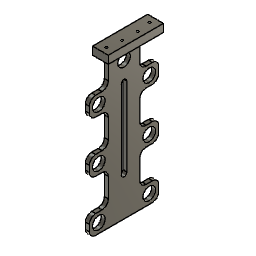
Riel Versión 3 v1 (Autodesk Fusion 360 design; units mm, degrees)
Autodesk Fusion 360 part; units mm, degrees
sketch "Boceto1" plane through (0, 0, 0) normal (0, 0, 1) x (1, 0, 0)
  line L0 (0, 0) -> (60, 0)
  line L1 (60, 0) -> (60, 40)
  line L2 (60, 40) -> (0, 40)
  line L3 (0, 40) -> (0, 0)
  line L4 (0, 0) -> (0, 10)
  line L5 (0, 40) -> (0, 30)
  line L6 (0, 30) -> (60, 30)
  line L7 (0, 10) -> (60, 10)
  line L8 (0, 30) -> (10, 30)
  line L9 (10, 40) -> (10, 0)
  line L10 (60, 40) -> (50, 40)
  line L11 (50, 40) -> (50, 0)
  circle A0 centre (5, 35) radius 2.5
  circle A1 centre (5, 5) radius 2.5
  circle A2 centre (55, 35) radius 2.5
  circle A3 centre (55, 5) radius 2.5
  line L12 (10, 10) -> (10, 9)
  line L13 (10, 9) -> (50, 9)
  line L14 (50, 30) -> (50, 31)
  line L15 (50, 31) -> (10, 31)
  line L16 (10, 0) -> (19, 0)
  line L17 (19, 9) -> (19, 0)
  line L18 (50, 0) -> (41, 0)
  line L19 (41, 0) -> (41, 9)
  line L20 (50, 31) -> (41, 31)
  line L21 (41, 31) -> (41, 40)
  line L22 (10, 31) -> (19, 31)
  line L23 (19, 31) -> (19, 40)
  line L24 (19, 9) -> (10, 0)
  line L25 (10, 9) -> (19, 0)
  circle A4 centre (14.5, 4.5) radius 2.5
  line L26 (19, 31) -> (10, 40)
  line L27 (50, 31) -> (41, 40)
  line L28 (50, 0) -> (41, 9)
  line L29 (50, 9) -> (41, 0)
  line L30 (50, 40) -> (41, 31)
  line L31 (19, 40) -> (10, 31)
  circle A5 centre (14.5, 35.5) radius 2.5
  circle A6 centre (45.5, 35.5) radius 2.5
  circle A7 centre (45.5, 4.5) radius 2.5
  line L32 (10, 9) -> (15, 9)
  line L33 (15, 9) -> (15, 31)
  line L34 (50, 9) -> (45, 9)
  line L35 (45, 9) -> (45, 31)
  dimension "d1" = 60
  dimension "d2" = 40
  dimension "d3" = 10
  dimension "d4" = 10
  dimension "d5" = 5
  dimension "d6" = 5
  dimension "d7" = 5
  dimension "d8" = 5
  dimension "d9" = 5
  dimension "d10" = 5
  dimension "d11" = 5
  dimension "d12" = 5
  constraint coincident L0.start L3.end
  constraint horizontal L0
  constraint perpendicular L0 L1
  constraint perpendicular L1 L2
  constraint perpendicular L0 L3
  constraint perpendicular L0 L4
  constraint perpendicular L2 L5
  constraint coincident L1 L6.end
  constraint perpendicular L1 L6
  constraint coincident L1 L7.end
  constraint perpendicular L1 L7
  constraint coincident L6 L8.end
  constraint coincident L2 L9.start
  constraint coincident L0 L9.end
  constraint perpendicular L0 L9
  constraint coincident L2 L10.end
  constraint perpendicular L7 L11
  constraint coincident L9 L12.start
  constraint coincident L7 L12.start
  constraint coincident L9 L12.end
  constraint coincident L11 L13.end
  constraint perpendicular L11 L13
  constraint coincident L11 L14.start
  constraint coincident L6 L14.start
  constraint coincident L11 L14.end
  constraint perpendicular L6 L14
  constraint coincident L9 L15.end
  constraint perpendicular L9 L15
  constraint coincident L0 L16.end
  constraint coincident L13 L17.start
  constraint perpendicular L16 L17
  constraint coincident L0 L18.end
  constraint perpendicular L11 L18
  constraint coincident L13 L19.end
  constraint perpendicular L13 L19
  constraint coincident L15 L20.end
  constraint coincident L2 L21.end
  constraint perpendicular L2 L21
  constraint coincident L15 L22.end
  constraint coincident L2 L23.end
  constraint perpendicular L2 L23
  constraint perpendicular L24 L25
  constraint midpoint L25 A4.centre
  constraint parallel L26 L27
  constraint parallel L27 L28
  constraint perpendicular L28 L29
  constraint midpoint L26 A5.centre
  constraint midpoint L30 A6.centre
  constraint midpoint L28 A7.centre
  constraint coincident L13 L32.end
  constraint perpendicular L9 L32
  constraint coincident L22 L33.end
  constraint coincident L13 L34.end
  constraint perpendicular L11 L34
  constraint coincident L20 L35.end
  measures "d1" distance of L0.start L0.end
  measures "d2" distance of L0.end L1.end
  measures "d3" distance of L0.start L4.end
  measures "d4" distance of L2.end L5.end
  measures "d5" diameter of A0
  measures "d6" diameter of A1
  measures "d7" diameter of A2
  measures "d8" diameter of A3
  measures "d9" diameter of A4
  measures "d10" diameter of A5
  measures "d11" diameter of A6
  measures "d12" diameter of A7
extrude "Extruir3" add sketch "Boceto1" along normal blind 20 contours L0 L3 L4 L7 L9 L12 | L0 L16 L24 L25 A4 | L9 L24 L25 A4 | L3 L6 L7 L8 L9 | L0 L13 L17 L19 | L17 L24 L25 A4 | L7 L9 L12 L13 L32 L33 | L13 L24 L25 A4 L32 | L2 L3 L5 L6 L8 L9 | L6 L7 L9 L33 | L0 L18 L28 L29 A7 | L19 L28 L29 A7 | L6 L9 L15 L22 L33 | L0 L1 L7 L11 | L11 L28 L29 A7 | L13 L28 L29 A7 L34 | L9 L26 L31 A5 | L2 L26 L31 A5 | L15 L22 L26 L31 A5 | L6 L7 L11 L35 | L7 L11 L13 L34 L35 | L2 L15 L21 L23 | L23 L26 L31 A5 | L6 L11 L14 L15 L20 L35 | L1 L6 L7 L11 | L21 L27 L30 A6 | L2 L27 L30 A6 | L1 L2 L6 L10 L11 L14 | L15 L20 L27 L30 A6 | L11 L27 L30 A6 | A0 | A1 | A2 | A3 makes body 1
extrude "Extruir4" add sketch "Boceto1" against normal blind 25 contours L0 L16 L24 L25 A4 | L9 L24 L25 A4 | L17 L24 L25 A4 | L7 L9 L12 L13 L32 L33 | L13 L24 L25 A4 L32 | L6 L7 L9 L33 | L0 L18 L28 L29 A7 | L19 L28 L29 A7 | L6 L9 L15 L22 L33 | L11 L28 L29 A7 | L13 L28 L29 A7 L34 | L9 L26 L31 A5 | L2 L26 L31 A5 | L15 L22 L26 L31 A5 | L6 L7 L11 L35 | L7 L11 L13 L34 L35 | L23 L26 L31 A5 | L6 L11 L14 L15 L20 L35 | L21 L27 L30 A6 | L2 L27 L30 A6 | L15 L20 L27 L30 A6 | L11 L27 L30 A6 bodies 1
sketch "Boceto2" plane through (15, 0, 0) normal (1, 0, 0) x (0, 1, 0)
  line L0 (31, -25) -> (31, 20)
  line L1 (31, 20) -> (9, 20)
  line L2 (9, 20) -> (9, -25)
  line L3 (9, -25) -> (31, -25)
  line L4 (20, 20) -> (20, -2)
  line L5 (20, -2) -> (20, -10)
  circle A0 centre (20, -10) radius 8
  dimension "d21" = 22
  dimension "d22" = 8
  constraint midpoint L1 L4.start
  constraint perpendicular L1 L4
  constraint parallel L4 L5
  constraint coincident L5.end A0.centre
  constraint coincident L4.end A0
  measures "d21" distance of L4.start L4.end
  measures "d22" distance of L4.end L5.end
extrude "Extruir5" cut sketch "Boceto2" along normal mid plane 100 contours A0 bodies 1
ref_plane "PlanoDeObra1" through (30, 20, 10) normal (-1, 0, 0) x (0, -1, 0)
split "Dividir1" by plane through (30, 20, 10) normal (-1, 0, 0) bodies 1 makes body 2 at (4.2441, 15.4226, 20)
extrude "Extruir6" cut 2 faces at (37.3333, 34, 0) (33.6667, 6, 0) along direction (0, 0, -1) up to surface end surface through (0, 0, 20) normal (0, 0, 1) offset 0 on bodies 1 bodies 1
extrude "Extruir7" cut 1 faces at (53.3333, 26.6667, 0) along direction (0, 0, 1) blind 5 on bodies 1 bodies 1
sketch "Boceto3" plane through (0, 0, -25) normal (0, 0, -1) x (1, 0, 0)
  circle A0 centre (45.5, -4.5) radius 2.5
  circle A1 centre (45.5, -35.5) radius 2.5
  line L0 (50, -40) -> (50, 0)
  line L1 (50, 0) -> (41, 0)
  line L2 (41, 0) -> (41, -9)
  line L3 (41, -9) -> (45, -9)
  line L4 (45, -9) -> (45, -31)
  line L5 (45, -31) -> (41, -31)
  line L6 (41, -31) -> (41, -40)
  line L7 (41, -40) -> (50, -40)
  line L8 (45, -9) -> (50, -9)
  line L9 (45, -31) -> (50, -31)
  constraint coincident L3.end L4.start
  constraint coincident L0 L8.end
  constraint perpendicular L0 L8
  constraint coincident L4.end L5.start
  constraint coincident L0 L9.end
  constraint perpendicular L0 L9
extrude "Extruir8" add sketch "Boceto3" along normal blind 160 contours L0 L5 L6 L7 L9 | L0 L1 L2 L3 L8 bodies 1
extrude "Extruir9" add 1 faces at (45, 19.8007, 12.6592) along direction (-1, 0, 0) up to surface (4 mm away) on bodies 1 bodies 1
sketch "Boceto4" plane through (41, 0, 0) normal (-1, 0, 0) x (0, -1, 0)
  circle A0 centre (-20, -10) radius 8
  line L0 (-9, -25) -> (-9, -185)
  line L1 (-9, -185) -> (0, -185)
  line L2 (0, -185) -> (0, 20)
  line L3 (0, 20) -> (-40, 20)
  line L4 (-40, 20) -> (-40, -25)
  line L5 (-40, -25) -> (-40, -185)
  line L6 (-40, -185) -> (-31, -185)
  line L7 (-31, -185) -> (-31, -25)
  line L8 (-31, -25) -> (-9, -25)
  line L9 (-9, -185) -> (-31, -185)
  line L10 (-20, -60) -> (-17.5, -60)
  line L11 (-20, -60) -> (-17.5, -60)
  line L12 (0, 20) -> (0, -110)
  line L13 (0, -110) -> (-40, -110)
  line L14 (-17.5, -110) -> (-17.5, -135)
  line L15 (-22.5, -110) -> (-22.5, -135)
  line L16 (-22.5, -135) -> (-20, -135)
  line L17 (-20, -135) -> (-17.5, -135)
  circle A1 centre (-20, -135) radius 2.5
  line L18 (-20, -25) -> (-20, -32.5)
  line L19 (-20, -32.5) -> (-20, -35)
  circle A2 centre (-20, -35) radius 2.5
  line L20 (-17.5, -35) -> (-17.5, -110)
  line L21 (-22.5, -110) -> (-22.5, -35)
  dimension "d41" = 130
  dimension "d43" = 25
  dimension "d44" = 7.5
  dimension "d45" = 2.5
  constraint coincident L0.end L1.start
  constraint coincident L6.end L7.start
  constraint coincident L2.end L3.start
  constraint perpendicular L3 L12
  constraint coincident L5 L13.end
  constraint perpendicular L5 L13
  constraint coincident L13 L14.start
  constraint perpendicular L13 L14
  constraint coincident L13 L15.start
  constraint perpendicular L15 L16
  constraint coincident L16.end L17.start
  constraint coincident L14.end A1
  constraint midpoint L8 L18.start
  constraint perpendicular L8 L18
  constraint parallel L18 L19
  constraint coincident L19.end A2.centre
  constraint coincident L18.end A2
  constraint coincident A2 L20.start
  constraint tangent A2 L20
  constraint coincident A2 L21.end
  constraint tangent A2 L21
  constraint perpendicular L8 L21
  measures "d41" distance of L2.end L12.end
  measures "d43" distance of L14.start L14.end
  measures "d44" distance of L18.start L18.end
  measures "d45" distance of L18.end L19.end
extrude "Extruir10" add sketch "Boceto4" against normal up to surface (9 mm away) contours L0 L8 L13 L18 A2 L20 | L0 L7 L9 L13 L14 L15 A1 | L7 L8 L13 L18 A2 L21 bodies 1
sketch "Boceto5" plane through (50, 0, 0) normal (1, 0, 0) x (0, 1, 0)
  line L0 (22.5, -35) -> (22.5, -135)
  arc A0 (17.5, -135) -> (22.5, -135) centre (20, -135) ccw
  line L1 (17.5, -135) -> (17.5, -35)
  arc A1 (22.5, -35) -> (17.5, -35) centre (20, -35) ccw
  circle A2 centre (20, -10) radius 8
  line L2 (0, 5) -> (0, -185)
  line L3 (0, -185) -> (40, -185)
  line L4 (40, -185) -> (40, -25)
  line L5 (40, -25) -> (40, 5)
  line L6 (40, 5) -> (0, 5)
  circle A3 centre (20, -35) radius 3.5
  circle A4 centre (20, -135) radius 3.5
  line L7 (23.5, -135) -> (23.5, -35)
  line L8 (16.5, -35) -> (16.5, -135)
  dimension "d46" = 7
  dimension "d47" = 7
  constraint concentric A1 A3
  constraint concentric A0 A4
  constraint coincident A4 L7.start
  constraint coincident A3 L7.end
  constraint tangent A3 L7
  constraint parallel L0 L7
  constraint coincident A3 L8.start
  constraint coincident A4 L8.end
  constraint tangent A4 L8
  constraint parallel L1 L8
  measures "d46" diameter of A3
  measures "d47" diameter of A4
extrude "Extruir11" cut sketch "Boceto5" against normal blind 50 contours L0 L1 A1 A3 | L0 A3 A4 L7 | L0 A0 L1 A4 | L1 A3 A4 L8 picked at (23.1443, -34.7019) picked at (16.8557, -135.2981) bodies 1
sketch "Boceto6" plane through (0, 0, 20) normal (0, 0, 1) x (-1, 0, 0)
  circle A0 centre (-45.5, -35.5) radius 2.5
  circle A1 centre (-45.5, -4.5) radius 2.5
  line L0 (-41, -40) -> (-41, 0)
  line L1 (-41, 0) -> (-60, 0)
  line L2 (-60, 0) -> (-60, -40)
  line L3 (-60, -40) -> (-41, -40)
  circle A2 centre (-45.5, -4.5) radius 2.5
  circle A3 centre (-45.5, -35.5) radius 2.5
  constraint concentric A1 A2
  constraint concentric A0 A3
extrude "Extruir12" add sketch "Boceto6" against normal up to surface (205 mm away) contours A0 A3 | A1 A2 bodies 1
extrude "Extruir13" cut 1 faces at (50, 19.9128, -169.4967) along direction (-1, 0, 0) blind 4 on bodies 1 bodies 1
extrude "Extruir14" cut 1 faces at (50.6667, 13.3333, 5) along direction (0, 0, 1) blind 5 on bodies 1 bodies 1
extrude "Extruir15" add 1 faces at (60, 13.3333, 13.3333) along direction (1, 0, 0) blind 1 on bodies 1 bodies 1
sketch "Boceto7" plane through (0, 40, 0) normal (0, 1, 0) x (-1, 0, 0)
  line L0 (-46, 10) -> (-46, -25)
  line L1 (-46, -25) -> (-41, -25)
  line L2 (-41, -25) -> (-41, 20)
  line L3 (-41, 20) -> (-61, 20)
  line L4 (-61, 20) -> (-61, 10)
  line L5 (-61, 10) -> (-46, 10)
  line L6 (-46, 10) -> (-41, 10)
  constraint coincident L0.start L5.end
  constraint coincident L2 L6.end
  constraint perpendicular L2 L6
extrude "Extruir16" add sketch "Boceto7" along normal blind 15 contours L2 L3 L4 L5 L6 bodies 1
sketch "Boceto8" plane through (0, 0, 0) normal (0, -1, 0) x (1, 0, 0)
  line L0 (46, -185) -> (46, 10)
  line L1 (46, 10) -> (61, 10)
  line L2 (61, 10) -> (61, 20)
  line L3 (61, 20) -> (41, 20)
  line L4 (41, 20) -> (41, -185)
  line L5 (41, -185) -> (46, -185)
  line L6 (46, 10) -> (41, 10)
  constraint coincident L0.end L1.start
  constraint coincident L4 L6.end
  constraint perpendicular L4 L6
extrude "Extruir17" add sketch "Boceto8" along normal blind 15 contours L1 L2 L3 L4 L6 bodies 1
sketch "Boceto9" plane through (46, 0, 0) normal (1, 0, 0) x (0, 1, 0)
  arc A0 (16.5, -135) -> (23.5, -135) centre (20, -135) ccw
  line L0 (16.5, -135) -> (16.5, -35)
  arc A1 (23.5, -35) -> (16.5, -35) centre (20, -35) ccw
  line L1 (23.5, -35) -> (23.5, -135)
  circle A2 centre (20, -10) radius 8
  line L2 (0, 10) -> (0, -185)
  line L3 (0, -185) -> (40, -185)
  line L4 (40, -185) -> (40, -25)
  line L5 (40, -25) -> (40, 10)
  line L6 (40, 10) -> (0, 10)
  line L7 (40, -185) -> (50, -185)
  line L8 (50, -185) -> (50, -175)
  line L9 (50, -175) -> (40, -175)
  line L10 (50, -128.3333) -> (40, -128.3333)
  line L11 (40, -138.3333) -> (50, -138.3333)
  line L12 (50, -138.3333) -> (50, -128.3333)
  line L13 (50, -81.6667) -> (40, -81.6667)
  line L14 (40, -91.6667) -> (50, -91.6667)
  line L15 (50, -91.6667) -> (50, -81.6667)
  line L16 (50, -35) -> (40, -35)
  line L17 (40, -45) -> (50, -45)
  line L18 (50, -45) -> (50, -35)
  dimension "d64" = 0
  dimension "d65" = 140
  constraint coincident L3.end L4.start
  constraint perpendicular L4 L7
  constraint perpendicular L3 L8
  constraint coincident L4 L9.end
  constraint perpendicular L4 L9
extrude "Extruir18" add sketch "Boceto9" against normal up to surface (5 mm away) contours L4 L7 L8 L9 | L4 L16 L17 L18 | L4 L10 L11 L12 | L4 L13 L14 L15 bodies 1
ref_plane "PlanoDeObra2" through (51, 20, 15) normal (0, 1, 0) x (0, 0, 1)
mirror "Simetría1" about plane through (51, 20, 15) normal (0, 1, 0) of bodies 1 merged
sketch "Boceto10" plane through (0, 0, 10) normal (0, 0, -1) x (1, 0, 0)
  line L0 (61, -55) -> (61, 15)
  line L1 (61, 15) -> (41, 15)
  line L2 (41, 15) -> (41, 0)
  line L3 (41, 0) -> (46, 0)
  line L4 (46, 0) -> (46, -40)
  line L5 (46, -40) -> (41, -40)
  line L6 (41, -40) -> (41, -55)
  line L7 (41, -55) -> (61, -55)
  line L8 (41, -55) -> (41, -40)
  line L9 (41, -40) -> (61, -40)
  line L10 (61, 15) -> (61, 0)
  line L11 (61, 0) -> (41, 0)
  line L12 (61, -40) -> (41, -55)
  circle A0 centre (51, -47.5) radius 1.5
  line L13 (61, 0) -> (41, 15)
  circle A1 centre (51, 7.5) radius 1.5
  line L14 (61, 0) -> (61, -40)
  line L15 (61, -20) -> (46, -20)
  line L16 (53.5, -20) -> (53.5, -40)
  line L17 (53.5, -20) -> (53.5, 0)
  circle A2 centre (53.5, -30) radius 1.5
  circle A3 centre (53.5, -10) radius 1.5
  dimension "d71" = 3
  dimension "d72" = 3
  dimension "d73" = 3
  dimension "d74" = 3
  constraint coincident L6.end L7.start
  constraint coincident L5.end L6.start
  constraint coincident L0 L9.end
  constraint perpendicular L0 L9
  constraint coincident L0.end L1.start
  constraint coincident L0 L10.end
  constraint perpendicular L1 L10
  constraint coincident L2.end L3.start
  constraint perpendicular L2 L11
  constraint midpoint L12 A0.centre
  constraint coincident L1.end L2.start
  constraint midpoint L13 A1.centre
  constraint midpoint L14 L15.start
  constraint midpoint L4 L15.end
  constraint midpoint L15 L16.start
  constraint coincident L9 L16.end
  constraint perpendicular L9 L16
  constraint coincident L11 L17.end
  constraint perpendicular L11 L17
  constraint midpoint L16 A2.centre
  constraint midpoint L17 A3.centre
  measures "d71" diameter of A0
  measures "d72" diameter of A1
  measures "d73" diameter of A2
  measures "d74" diameter of A3
extrude "Extruir19" cut sketch "Boceto10" against normal up to surface (10 mm away) contours L12 A0 | L12 A0 | L16 A2 | L16 A2 | L13 A1 | L13 A1 | L17 A3 | L17 A3 bodies 1
extrude "Extruir20" cut 1 faces at (42.6667, -6.6667, -35) along direction (0, 0, -1) up to surface (150 mm away) on bodies 1 bodies 1
extrude "Extruir21" cut 1 faces at (42.6667, 46.6667, -35) along direction (0, 0, -1) up to surface (150 mm away) on bodies 1 bodies 1
sketch "Boceto11" plane through (41, 0, 0) normal (-1, 0, 0) x (0, -1, 0)
  circle A0 centre (-20, -10) radius 8
  arc A1 (-23.5, -135) -> (-16.5, -135) centre (-20, -135) ccw
  line L0 (-23.5, -135) -> (-23.5, -35)
  arc A2 (-16.5, -35) -> (-23.5, -35) centre (-20, -35) ccw
  line L1 (-16.5, -35) -> (-16.5, -135)
  line L2 (-40, -25) -> (-40, -185)
  line L3 (-40, -185) -> (0, -185)
  line L4 (0, -185) -> (0, 10)
  line L5 (0, 10) -> (15, 10)
  line L6 (15, 10) -> (15, 20)
  line L7 (15, 20) -> (-55, 20)
  line L8 (-55, 20) -> (-55, 10)
  line L9 (-55, 10) -> (-40, 10)
  line L10 (-40, 10) -> (-40, -25)
  line L11 (-40, -185) -> (-56, -185)
  line L12 (-64, -177) -> (-64, -169)
  line L13 (-56, -161) -> (-40, -161)
  line L14 (-64, -185) -> (-40, -161)
  circle A3 centre (-52, -173) radius 8
  line L15 (0, -185) -> (16, -185)
  line L16 (24, -177) -> (24, -169)
  line L17 (16, -161) -> (0, -161)
  line L18 (0, -161) -> (24, -185)
  circle A4 centre (12, -173) radius 8
  arc A5 (16, -185) -> (24, -177) centre (16, -177) ccw
  arc A6 (24, -169) -> (16, -161) centre (16, -169) ccw
  arc A7 (-64, -177) -> (-56, -185) centre (-56, -177) ccw
  arc A8 (-56, -161) -> (-64, -169) centre (-56, -169) ccw
  arc A9 (24, -104) -> (16, -96) centre (16, -104) ccw
  circle A10 centre (12, -108) radius 8
  arc A11 (16, -120) -> (24, -112) centre (16, -112) ccw
  line L19 (24, -112) -> (24, -104)
  line L20 (0, -120) -> (16, -120)
  line L21 (16, -96) -> (0, -96)
  line L22 (-64, -112) -> (-64, -104)
  arc A12 (-64, -112) -> (-56, -120) centre (-56, -112) ccw
  arc A13 (-56, -96) -> (-64, -104) centre (-56, -104) ccw
  line L23 (-40, -120) -> (-56, -120)
  circle A14 centre (-52, -108) radius 8
  line L24 (-56, -96) -> (-40, -96)
  arc A15 (24, -39) -> (16, -31) centre (16, -39) ccw
  circle A16 centre (12, -43) radius 8
  arc A17 (16, -55) -> (24, -47) centre (16, -47) ccw
  line L25 (24, -47) -> (24, -39)
  line L26 (0, -55) -> (16, -55)
  line L27 (16, -31) -> (0, -31)
  line L28 (-64, -47) -> (-64, -39)
  arc A18 (-64, -47) -> (-56, -55) centre (-56, -47) ccw
  arc A19 (-56, -31) -> (-64, -39) centre (-56, -39) ccw
  line L29 (-40, -55) -> (-56, -55)
  circle A20 centre (-52, -43) radius 8
  line L30 (-56, -31) -> (-40, -31)
  point P0 (-64, -161)
  point P1 (24, -161)
  point P2 (24, -120)
  point P3 (24, -96)
  point P4 (-64, -120)
  point P5 (-64, -96)
  point P6 (24, -55)
  point P7 (24, -31)
  point P8 (-64, -55)
  point P9 (-64, -31)
  dimension "d81" = 24
  dimension "d82" = 24
  dimension "d83" = 24
  dimension "d84" = 16
  dimension "d85" = 24
  dimension "d86" = 24
  dimension "d87" = 16
  dimension "d88" = 8
  dimension "d89" = 8
  dimension "d90" = 8
  dimension "d91" = 8
  dimension "d94" = 0
  dimension "d95" = 130
  constraint coincident L2.end L3.start
  constraint perpendicular L2 L11
  constraint perpendicular L11 L12
  constraint perpendicular L12 L13
  constraint midpoint L14 A3.centre
  constraint coincident L3.end L4.start
  constraint perpendicular L4 L15
  constraint perpendicular L15 L16
  constraint coincident L4 L17.end
  constraint perpendicular L4 L17
  constraint midpoint L18 A4.centre
  constraint coincident L18.end L15
  constraint coincident L18.end L16
  constraint tangent L15 A5
  constraint tangent L16 A5
  constraint coincident P1 L16
  constraint coincident P1 L17
  constraint tangent L16 A6
  constraint tangent L17 A6
  constraint coincident L14.start L11
  constraint coincident L14.start L12
  constraint tangent L11 A7
  constraint tangent L12 A7
  constraint coincident P0 L13
  constraint coincident P0 L12
  constraint tangent L13 A8
  constraint tangent L12 A8
  measures "d81" distance of L2.end L14.start
  measures "d82" distance of L14.start P0
  measures "d83" distance of P0 L13.end
  measures "d84" diameter of A3
  measures "d85" distance of L3.end L18.end
  measures "d86" distance of L18.end P1
  measures "d87" diameter of A4
  measures "d88" radius of A5
  measures "d89" radius of A6
  measures "d90" radius of A7
  measures "d91" radius of A8
extrude "Extruir22" add sketch "Boceto11" against normal up to surface (5 mm away) contours L2 L28 A18 A19 L29 L30 | L2 L22 A12 A13 L23 L24 | L12 L13 L14 A3 A7 A8 | L2 L11 L14 A3 A7 | L4 L15 L18 A4 A5 | L4 A15 A17 L25 L26 L27 | L16 L17 L18 A4 A5 A6 | L4 A9 A11 L19 L20 L21 bodies 1
fillet "Empalme1" radius 8 10 edges at (43.5, 0, -161) (43.5, 40, -161) (43.5, 40, -120) (43.5, 0, -120) (43.5, 0, -96) (43.5, 40, -96) (43.5, 0, -55) (43.5, 40, -55) (43.5, 40, -31) (43.5, 0, -31) on bodies 1
hidden bodies 2
